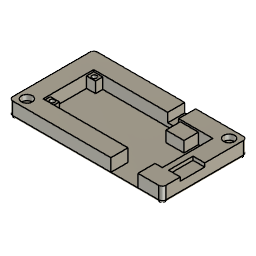
ASSEMBLY v9 (Autodesk Fusion 360 archive; units mm, degrees)
design "BOTTOM"
Autodesk Fusion 360 part; units mm, degrees
sketch "Sketch1" plane through (0, 0, 0) normal (0, 0, 1) x (1, 0, 0)
  line L0 (0, 0) -> (65, 0)
  line L1 (65, 0) -> (65, 27)
  line L2 (65, 27) -> (0, 27)
  line L3 (0, 27) -> (0, 0)
  line L4 (-10, -10) -> (75, -10)
  line L5 (75, -10) -> (75, 37)
  line L6 (75, 37) -> (-10, 37)
  line L7 (-10, 37) -> (-10, -10)
  dimension "d3" = 65
  dimension "d4" = 27
  dimension "d5" = 85
  dimension "d6" = 47
  dimension "d7" = 10
  dimension "d8" = 10
  constraint horizontal L0
  constraint vertical L1
  constraint horizontal L2
  constraint vertical L3
  constraint coincident L0.start L3.end
  constraint horizontal L4
  constraint vertical L5
  constraint horizontal L6
  constraint vertical L7
  measures "d3" distance of L1.end L2.end
  measures "d4" distance of L0.start L2.end
  measures "d5" distance of L5.end L6.end
  measures "d6" distance of L4.end L5.end
  measures "d7" distance of L2 L6
  measures "d8" distance of L1 L5
extrude "Extrude1" add sketch "Sketch1" along normal blind 2 contours L0 L1 L2 L3 | L4 L5 L6 L7
sketch "Sketch2" plane through (0, 0, 2) normal (0, 0, 1) x (-1, 0, 0)
  line L0 (10, -37) -> (10, 10)
  line L1 (10, 10) -> (-75, 10)
  line L2 (-75, 10) -> (-75, -37)
  line L3 (-75, -37) -> (10, -37)
  line L4 (-65.5, -27.5) -> (0.5, -27.5)
  line L5 (0.5, -27.5) -> (0.5, 0.5)
  line L6 (0.5, 0.5) -> (-65.5, 0.5)
  line L7 (-65.5, 0.5) -> (-65.5, -27.5)
  dimension "d19" = 66
  dimension "d20" = 28
  dimension "d21" = 9.5
  dimension "d22" = 9.5
  constraint horizontal L4
  constraint vertical L5
  constraint horizontal L6
  constraint vertical L7
  measures "d19" distance of L4.start L4.end
  measures "d20" distance of L4.start L6.end
  measures "d21" distance of L3 L4
  measures "d22" distance of L2 L7
extrude "Extrude3" add sketch "Sketch2" along normal blind 7
sketch "Sketch3" plane through (0, 0, 2) normal (0, 0, 1) x (-1, 0, 0)
  circle A0 centre (-2.1, -25.25) radius 1.1
  line L0 (0.5, -27.5) -> (0.5, 0.5)
  line L1 (-65.5, -27.5) -> (0.5, -27.5)
  circle A1 centre (-2.1, -1.75) radius 1.1
  line L2 (0.5, 0.5) -> (-65.5, 0.5)
  dimension "d25" = 2.2
  dimension "d26" = 2.6
  dimension "d27" = 2.25
  dimension "d28" = 2.2
  dimension "d29" = 2.25
  dimension "d30" = 2.6
  measures "d25" diameter of A0
  measures "d26" distance of A0.centre L0
  measures "d27" distance of A0.centre L1
  measures "d28" diameter of A1
  measures "d29" distance of A1.centre L2
  measures "d30" distance of L0 A1.centre
extrude "Extrude4" cut sketch "Sketch3" against normal blind 3
sketch "Sketch4" plane through (0, 0, 9) normal (0, 0, 1) x (-1, 0, 0)
  line L0 (-65.5, -27.5) -> (-65.5, 0.5)
  line L1 (-65.5, 0.5) -> (0.5, 0.5)
  line L2 (0.5, 0.5) -> (0.5, -27.5)
  line L3 (0.5, -27.5) -> (-65.5, -27.5)
  line L4 (-75, -37) -> (10, -37)
  line L5 (10, -37) -> (10, 10)
  line L6 (10, 10) -> (-75, 10)
  line L7 (-75, 10) -> (-75, -37)
  line L8 (-46.5, -37) -> (-40.5, -37)
  line L9 (-40.5, -37) -> (-40.5, -27.5)
  line L10 (-40.5, -27.5) -> (-46.5, -27.5)
  line L11 (-46.5, -27.5) -> (-46.5, -37)
  line L12 (0.5, -27.5) -> (0.5, 0.5)
  line L13 (-65.5, 0.5) -> (-65.5, -27.5)
  dimension "d34" = 41
  dimension "d35" = 19
  constraint horizontal L8
  constraint vertical L9
  constraint horizontal L10
  constraint vertical L11
  constraint coincident L3 L9.end
  constraint coincident L4 L8.start
  measures "d34" distance of L9 L12
  measures "d35" distance of L11 L13
extrude "Extrude5" cut sketch "Sketch4" against normal blind 5 contours L3 L4 L8 L9 L10 L11
sketch "Sketch7" plane through (0, 0, 9) normal (0, 0, 1) x (-1, 0, 0)
  line L0 (-46.5, -37) -> (-46.5, -27.5)
  line L1 (-46.5, -27.5) -> (-65.5, -27.5)
  line L2 (-65.5, -27.5) -> (-65.5, 0.5)
  line L3 (-65.5, 0.5) -> (0.5, 0.5)
  line L4 (0.5, 0.5) -> (0.5, -27.5)
  line L5 (0.5, -27.5) -> (-40.5, -27.5)
  line L6 (-40.5, -27.5) -> (-40.5, -37)
  line L7 (-40.5, -37) -> (10, -37)
  line L8 (10, -37) -> (10, 10)
  line L9 (10, 10) -> (-75, 10)
  line L10 (-75, 10) -> (-75, -37)
  line L11 (-75, -37) -> (-46.5, -37)
  circle A0 centre (5, 5) radius 3
  circle A1 centre (-70, -32) radius 3
  dimension "d52" = 6
  dimension "d53" = 5
  dimension "d54" = 5
  dimension "d55" = 6
  dimension "d56" = 5
  dimension "d57" = 5
  measures "d52" diameter of A0
  measures "d53" distance of L8 A0.centre
  measures "d54" distance of L9 A0.centre
  measures "d55" diameter of A1
  measures "d56" distance of L11 A1.centre
  measures "d57" distance of L10 A1.centre
extrude "Extrude7" cut sketch "Sketch7" against normal blind 3 contours A0 | A1
sketch "Sketch8" plane through (0, 0, 9) normal (0, 0, 1) x (-1, 0, 0)
  circle A0 centre (5, 5) radius 3
  circle A1 centre (-70, -32) radius 3
  line L0 (-46.5, -37) -> (-46.5, -27.5)
  line L1 (-46.5, -27.5) -> (-65.5, -27.5)
  line L2 (-65.5, -27.5) -> (-65.5, 0.5)
  line L3 (-65.5, 0.5) -> (0.5, 0.5)
  line L4 (0.5, 0.5) -> (0.5, -27.5)
  line L5 (0.5, -27.5) -> (-40.5, -27.5)
  line L6 (-40.5, -27.5) -> (-40.5, -37)
  line L7 (-40.5, -37) -> (10, -37)
  line L8 (10, -37) -> (10, 10)
  line L9 (10, 10) -> (-75, 10)
  line L10 (-75, 10) -> (-75, -37)
  line L11 (-75, -37) -> (-46.5, -37)
  line L12 (-46.5, 0.5) -> (-61.5, 0.5)
  line L13 (-61.5, 0.5) -> (-61.5, 10)
  line L14 (-61.5, 10) -> (-46.5, 10)
  line L15 (-46.5, 10) -> (-46.5, 0.5)
  line L16 (0.5, -27.5) -> (0.5, 0.5)
  line L17 (-65.5, 0.5) -> (-65.5, -27.5)
  dimension "d61" = 47
  dimension "d62" = 4
  constraint horizontal L12
  constraint vertical L13
  constraint horizontal L14
  constraint vertical L15
  constraint coincident L9 L13.end
  constraint coincident L3 L12.start
  measures "d61" distance of L15 L16
  measures "d62" distance of L13 L17
extrude "Extrude8" cut sketch "Sketch8" against normal blind 7 contours L3 L9 L12 L13 L14 L15
fillet "Fillet1" radius 2 4 edges at (-10, -10, 4.5) (75, -10, 4.5) (75, 37, 4.5) (-10, 37, 4.5)
sketch "Sketch9" plane through (0, 0, 9) normal (0, 0, 1) x (-1, 0, 0)
  arc A0 (-75, -35) -> (-73, -37) centre (-73, -35) ccw
  line L0 (-73, -37) -> (-46.5, -37)
  line L1 (-46.5, -37) -> (-46.5, -27.5)
  line L2 (-46.5, -27.5) -> (-65.5, -27.5)
  line L3 (-65.5, -27.5) -> (-65.5, 0.5)
  line L4 (-65.5, 0.5) -> (-61.5, 0.5)
  line L5 (-61.5, 0.5) -> (-61.5, 10)
  line L6 (-61.5, 10) -> (-73, 10)
  arc A1 (-73, 10) -> (-75, 8) centre (-73, 8) ccw
  line L7 (-75, 8) -> (-75, -35)
  circle A2 centre (-70, -32) radius 3
  line L8 (-75, 0) -> (-68.5, 0)
  line L9 (-68.5, 0) -> (-68.5, -13.5)
  line L10 (-68.5, -13.5) -> (-75, -13.5)
  line L11 (-75, -13.5) -> (-75, 0)
  line L12 (-65.5, 0.5) -> (-65.5, -27.5)
  dimension "d67" = 10
  dimension "d68" = 3
  dimension "d69" = 13.5
  constraint horizontal L8
  constraint vertical L9
  constraint horizontal L10
  constraint vertical L11
  constraint coincident L7 L8.start
  measures "d67" distance of L6 L8
  measures "d68" distance of L9 L12
  measures "d69" distance of L8.end L9.end
extrude "Extrude9" cut sketch "Sketch9" against normal blind 2 contours L7 L8 L9 L10 L11
sketch "Sketch10" plane through (0, 0, 0) normal (0, 0, -1) x (1, 0, 0)
  arc A0 (-10, -35) -> (-8, -37) centre (-8, -35) ccw
  line L0 (-8, -37) -> (73, -37)
  arc A1 (73, -37) -> (75, -35) centre (73, -35) ccw
  line L1 (75, -35) -> (75, 8)
  arc A2 (75, 8) -> (73, 10) centre (73, 8) ccw
  line L2 (73, 10) -> (-8, 10)
  arc A3 (-8, 10) -> (-10, 8) centre (-8, 8) ccw
  line L3 (-10, 8) -> (-10, -35)
  circle A4 centre (2.1, -25.25) radius 1.1
  circle A5 centre (2.1, -1.75) radius 1.1
  line L4 (-0.5, 0.5) -> (65.5, 0.5)
  line L5 (-0.5, -27.5) -> (-0.5, 0.5)
  circle A6 centre (2.1, -25.25) radius 1.1
  circle A7 centre (2.1, -1.75) radius 1.1
  dimension "d75" = 2.2
  constraint concentric A4 A6
  constraint concentric A5 A7
  measures "d75" diameter of A6
hole "Hole1" at (2.1, 2, 0) at (2.1, 25.25, 0) direction (0, 0, 1) diameter 2.6 depth 14 tip angle 180 countersink diameter 4.4 countersink angle 90
sketch "Sketch11" plane through (0, 0, 2) normal (0, 0, 1) x (-1, 0, 0)
  line L0 (-65.5, -27.5) -> (0.5, -27.5)
  line L1 (0.5, -27.5) -> (0.5, 0.5)
  line L2 (0.5, 0.5) -> (-46.5, 0.5)
  line L3 (-46.5, 0.5) -> (-46.5, 10)
  line L4 (-46.5, 10) -> (-61.5, 10)
  line L5 (-61.5, 10) -> (-61.5, 0.5)
  line L6 (-61.5, 0.5) -> (-65.5, 0.5)
  line L7 (-65.5, 0.5) -> (-65.5, -27.5)
  arc A0 (-2.8161, -0.915) -> (-1.3839, -0.915) centre (-2.1, -2) ccw
  arc A1 (-1.3839, -0.915) -> (-2.8161, -0.915) centre (-2.1, -1.75) ccw
  circle A2 centre (-2.1, -25.25) radius 1.3
  line L8 (0.5, -27.5) -> (-4.5, -27.5)
  line L9 (-4.5, -27.5) -> (-4.5, -23.5)
  line L10 (-4.5, -23.5) -> (0.5, -23.5)
  line L11 (0.5, -23.5) -> (0.5, -27.5)
  line L12 (0.5, 0.5) -> (-4.5, 0.5)
  line L13 (-4.5, 0.5) -> (-4.5, -3.5)
  line L14 (-4.5, -3.5) -> (0.5, -3.5)
  line L15 (0.5, -3.5) -> (0.5, 0.5)
  dimension "d81" = 5
  dimension "d82" = 4
  dimension "d83" = 5
  dimension "d84" = 4
  constraint horizontal L8
  constraint vertical L9
  constraint horizontal L10
  constraint vertical L11
  constraint coincident L0.end L1.start
  constraint horizontal L12
  constraint vertical L13
  constraint horizontal L14
  constraint vertical L15
  constraint coincident L1.end L2.start
  measures "d81" distance of L0.end L8.end
  measures "d82" distance of L0.end L10.end
  measures "d83" distance of L1.end L12.end
  measures "d84" distance of L1.end L14.end
extrude "Extrude10" add sketch "Sketch11" along normal blind 6 contours L0 L1 L8 L9 L10 L11 | L1 L2 L12 L13 L14 L15
sketch "Sketch12" plane through (0, 0, 2) normal (0, 0, 1) x (-1, 0, 0)
  line L0 (-4.5, -27.5) -> (-4.5, -23.5)
  line L1 (-4.5, -23.5) -> (0.5, -23.5)
  line L2 (0.5, -23.5) -> (0.5, -3.5)
  line L3 (0.5, -3.5) -> (-4.5, -3.5)
  line L4 (-4.5, -3.5) -> (-4.5, 0.5)
  line L5 (-4.5, 0.5) -> (-46.5, 0.5)
  line L6 (-46.5, 0.5) -> (-46.5, 10)
  line L7 (-46.5, 10) -> (-61.5, 10)
  line L8 (-61.5, 10) -> (-61.5, 0.5)
  line L9 (-61.5, 0.5) -> (-65.5, 0.5)
  line L10 (-65.5, 0.5) -> (-65.5, -27.5)
  line L11 (-65.5, -27.5) -> (-4.5, -27.5)
  line L12 (-47.5, -27.5) -> (-57.5, -27.5)
  line L13 (-57.5, -27.5) -> (-57.5, -19.5)
  line L14 (-57.5, -19.5) -> (-47.5, -19.5)
  line L15 (-47.5, -19.5) -> (-47.5, -27.5)
  dimension "d87" = 10
  dimension "d88" = 8
  dimension "d89" = 18
  constraint horizontal L12
  constraint vertical L13
  constraint horizontal L14
  constraint vertical L15
  constraint coincident L11 L12.start
  measures "d87" distance of L12.start L12.end
  measures "d88" distance of L12.start L14.end
  measures "d89" distance of L10 L15
extrude "Extrude11" add sketch "Sketch12" along normal blind 6 contours L11 L12 L13 L14 L15
fillet "Fillet2" radius 2 8 edges at (75, 13.5, 0) (74.4142, 36.4142, 0) (32.5, 37, 0) (-9.4142, 36.4142, 0) (-10, 13.5, 0) (-9.4142, -9.4142, 0) (32.5, -10, 0) (74.4142, -9.4142, 0)
